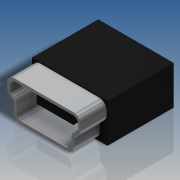
# Autodesk Inventor part: 11033-Black
Saved by Autodesk Inventor 2016 SP2 (Build 200236200, 236)
## iProperties
Created: 2015-08-21
Part Number: 11033-Black
Material: ABS Plastic
Document SubType Name: Modeling
Designer: D. Kohfeld
Mass: 0.214456 g
Surface Area: 4.85626 cm^2
Volume: 0.202317 cm^3
Density: 1.06 g/cm^3
Appearance: Black
Author: D. Kohfeld
Autodesk Inventor part; units mm, degrees
ref_plane "YZ Plane" through (0, 0, 0) normal (1, 0, 0) x (0, 1, 0)
ref_plane "XZ Plane" through (0, 0, 0) normal (0, 1, 0) x (-1, 0, 0)
ref_plane "XY Plane" through (0, 0, 0) normal (0, 0, 1) x (1, 0, 0)
imported_surface "0"
sketch "Sketch2" plane through (0, 0, 0) normal (0, 0, 1) x (1, 0, 0)
  line L0 (-4, 2) -> (4, 2)
  line L1 (4, 2) -> (4, -2)
  line L2 (4, -2) -> (-4, -2)
  line L3 (-4, -2) -> (-4, 2)
  point P0 (0, 0)
  point P1 (0, 2)
  point P2 (4, 0)
  dimension "d0" = 4
  dimension "d1" = 8
  constraints: 8 end point, 2 midpoint, 2 parallel, 1 horizontal, 1 horizontal alignment, 1 perpendicular, 1 vertical alignment
  measures "d0" distance of L0.end L1.end
  measures "d1" distance of L0.start L0.end
extrude "Extrusion1" add sketch "Sketch2" against normal blind 7.2
sketch "Sketch3" plane through (0, 0, 0) normal (0, 0, 1) x (1, 0, 0)
  line L0 (-4, 2) -> (4, 2) construction
  line L1 (-4, -2) -> (-4, 2) construction
  line L2 (4, -2) -> (-4, -2) construction
  line L3 (4, 2) -> (4, -2) construction
  line L4 (-3.2, 2) -> (3.2, 2)
  arc A0 (4, 1.2) -> (3.2, 2) centre (3.2, 1.2) ccw
  line L5 (4, 1.2) -> (4, 0.6928)
  arc A1 (3.6, 0) -> (4, 0.6928) centre (3.2, 0.6928) ccw
  line L6 (3.6, 0) -> (3.509, -0.0525)
  arc A2 (3.509, -0.0525) -> (3.259, -0.4856) centre (3.759, -0.4856) ccw
  line L7 (3.259, -0.4856) -> (3.259, -1.2)
  arc A3 (2.459, -2) -> (3.259, -1.2) centre (2.459, -1.2) ccw
  line L8 (2.459, -2) -> (-2.459, -2)
  arc A4 (-3.259, -1.2) -> (-2.459, -2) centre (-2.459, -1.2) ccw
  line L9 (-3.259, -1.2) -> (-3.259, -0.4856)
  arc A5 (-3.259, -0.4856) -> (-3.509, -0.0525) centre (-3.759, -0.4856) ccw
  line L10 (-3.509, -0.0525) -> (-3.6, 0)
  arc A6 (-4, 0.6928) -> (-3.6, 0) centre (-3.2, 0.6928) ccw
  line L11 (-4, 0.6928) -> (-4, 1.2)
  arc A7 (-3.2, 2) -> (-4, 1.2) centre (-3.2, 1.2) ccw
  line L12 (-3.45, 0.2598) -> (-3.359, 0.2073)
  arc A8 (-2.959, -0.4856) -> (-3.359, 0.2073) centre (-3.759, -0.4856) ccw
  line L13 (-2.959, -0.4856) -> (-2.959, -1.2)
  arc A9 (-2.959, -1.2) -> (-2.459, -1.7) centre (-2.459, -1.2) ccw
  line L14 (-2.459, -1.7) -> (2.459, -1.7)
  arc A10 (2.459, -1.7) -> (2.959, -1.2) centre (2.459, -1.2) ccw
  line L15 (2.959, -1.2) -> (2.959, -0.4856)
  arc A11 (3.359, 0.2073) -> (2.959, -0.4856) centre (3.759, -0.4856) ccw
  line L16 (3.359, 0.2073) -> (3.45, 0.2598)
  arc A12 (3.45, 0.2598) -> (3.7, 0.6928) centre (3.2, 0.6928) ccw
  line L17 (3.7, 0.6928) -> (3.7, 1.2)
  arc A13 (3.7, 1.2) -> (3.2, 1.7) centre (3.2, 1.2) ccw
  line L18 (3.2, 1.7) -> (-3.2, 1.7)
  arc A14 (-3.2, 1.7) -> (-3.7, 1.2) centre (-3.2, 1.2) ccw
  line L19 (-3.7, 1.2) -> (-3.7, 0.6928)
  arc A15 (-3.7, 0.6928) -> (-3.45, 0.2598) centre (-3.2, 0.6928) ccw
  line L20 (-2, 0.4) -> (2, 0.4)
  line L21 (2, 0.4) -> (2, -0.4)
  line L22 (2, -0.4) -> (-2, -0.4)
  line L23 (-2, -0.4) -> (-2, 0.4)
  point P0 (0, 0)
  point P1 (0, -2)
  point P2 (0, 0.4)
  point P3 (-2, 0)
  dimension "d4" = 6.518
  dimension "d5" = 0.8
  dimension "d8" = 0.3
  dimension "d9" = 60
  dimension "d12" = 4
  dimension "d13" = 0.8
  constraints: 42 end point, 32 point on circle, 17 tangent, 16 centre point, 7 equal radius, 6 point on line, 3 horizontal alignment, 3 midpoint, 3 vertical, 2 parallel, 2 vertical alignment, 1 equal length, 1 horizontal, 1 perpendicular, 15 other
  measures "d4" distance between parallel lines of L7 L9
  measures "d5" radius of A0
  measures "d8" distance between parallel lines of L0 L18
  measures "d9" angle of L1 L10
  measures "d12" distance of L20.start L20.end
  measures "d13" distance of L22.end L20.start
extrude "Extrusion2" add sketch "Sketch3" along normal blind 2.8 contours L4 A0 L5 A1 L6 A2 L7 A3 L8 A4 L9 A5 L10 A6 L11 A7
extrude "Extrusion3" add sketch "Sketch3" along normal blind 1.6 contours L20 L21 L22 L23
extrude "Extrusion4" cut sketch "Sketch3" against normal blind 3.6 contours A15 L19 A14 L18 A13 L17 A12 L16 A11 L15 A10 L14 A9 L13 A8 L12
sketch "Sketch4" plane through (-2, -0.4, 1.6) normal (0, -1, 0) x (1, 0, 0)
  line L0 (0, 0) -> (4, 0) projected
  line L1 (0, 0) -> (0, -5.2) projected
  line L2 (0, -5.2) -> (4, -5.2) projected
  line L3 (1.75, -0.2) -> (2.25, -0.2)
  line L4 (2.25, -0.2) -> (2.25, -5.2)
  line L5 (2.25, -5.2) -> (1.75, -5.2)
  line L6 (1.75, -5.2) -> (1.75, -0.2)
  line L7 (2.525, -0.2) -> (3.025, -0.2)
  line L8 (3.025, -0.2) -> (3.025, -5.2)
  line L9 (3.025, -5.2) -> (2.525, -5.2)
  line L10 (2.525, -5.2) -> (2.525, -0.2)
  line L11 (3.3, -0.2) -> (3.8, -0.2)
  line L12 (3.8, -0.2) -> (3.8, -5.2)
  line L13 (3.8, -5.2) -> (3.3, -5.2)
  line L14 (3.3, -5.2) -> (3.3, -0.2)
  line L15 (0.975, -0.2) -> (1.475, -0.2)
  line L16 (1.475, -0.2) -> (1.475, -5.2)
  line L17 (1.475, -5.2) -> (0.975, -5.2)
  line L18 (0.975, -5.2) -> (0.975, -0.2)
  line L19 (0.2, -0.2) -> (0.7, -0.2)
  line L20 (0.7, -0.2) -> (0.7, -5.2)
  line L21 (0.7, -5.2) -> (0.2, -5.2)
  line L22 (0.2, -5.2) -> (0.2, -0.2)
  line L23 (0.7, -0.2) -> (0.975, -0.2) construction
  line L24 (1.475, -0.2) -> (1.75, -0.2) construction
  line L25 (2.25, -0.2) -> (2.525, -0.2) construction
  line L26 (3.025, -0.2) -> (3.3, -0.2) construction
  line L27 (0.2, -0.2) -> (0.2, 0) construction
  line L28 (0.2, -0.2) -> (0, -0.2) construction
  point P0 (2, -1.6)
  point P1 (2, -0.2)
  dimension "d18" = 0.5
  dimension "d19" = 0.2
  constraints: 52 end point, 10 horizontal, 10 parallel, 8 equal length, 7 point on line, 5 perpendicular, 1 midpoint, 1 vertical, 1 vertical alignment
  measures "d18" distance of L3.start L3.end
  measures "d19" distance between parallel lines of L0 L19
extrude "Extrusion5" add sketch "Sketch4" along normal blind 0.01
sketch "Sketch5" plane through (0, 0, 0) normal (0, 0, 1) x (1, 0, 0)
  arc A0 (-3.2, 2) -> (-4, 1.2) centre (-3.2, 1.2) ccw projected
  line L0 (-4, 2) -> (-3.2, 2) projected
  line L1 (-4, 1.2) -> (-4, 2) projected
  arc A1 (4, 1.2) -> (3.2, 2) centre (3.2, 1.2) ccw projected
  line L2 (4, 2) -> (4, 1.2) projected
  line L3 (3.2, 2) -> (4, 2) projected
  arc A2 (2.459, -2) -> (3.259, -1.2) centre (2.459, -1.2) ccw projected
  line L4 (4, -2) -> (2.459, -2) projected
  line L5 (4, 0.6928) -> (4, -2) projected
  arc A3 (3.6, 0) -> (4, 0.6928) centre (3.2, 0.6928) ccw projected
  line L6 (3.6, 0) -> (3.509, -0.0525) projected
  arc A4 (3.509, -0.0525) -> (3.259, -0.4856) centre (3.759, -0.4856) ccw projected
  line L7 (3.259, -0.4856) -> (3.259, -1.2) projected
  line L8 (-4.1, 2.1) -> (4.1, 2.1)
  line L9 (4.1, 2.1) -> (4.1, -2.1)
  line L10 (4.1, -2.1) -> (-4.1, -2.1)
  line L11 (-4.1, -2.1) -> (-4.1, 2.1)
  line L12 (-4, 2) -> (4, 2)
  line L13 (4, 2) -> (4, -2)
  line L14 (4, -2) -> (-4, -2)
  line L15 (-4, -2) -> (-4, 2)
  point P0 (0, 0)
  point P1 (0, 2.1)
  point P2 (-4.1, 0)
  dimension "d22" = 0.1
  dimension "d24" = 0.1
  constraints: 16 end point, 4 parallel, 2 horizontal, 2 midpoint, 2 perpendicular, 1 horizontal alignment, 1 vertical alignment
  measures "d22" distance between parallel lines of L1 L11
  measures "d24" distance between parallel lines of L0 L8
extrude "Extrusion6" add sketch "Sketch5" against normal up to surface (7.2 mm away)
equation "\"d1\" = lu"
equation "\"d14\" = wall"
equation "\"d24\" = d22"
equation "\"lu\" = 8"
equation "\"wall\" = 1.6"
body "Solid1"
body "Srf1"
